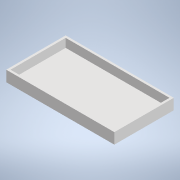
# Autodesk Inventor part: LowerHalf
Saved by Autodesk Inventor 2022 (Build 260153000, 153)
## iProperties
Created: 2023-09-02
Part Number: LowerHalf
Material: Generic
Document SubType Name: Modeling
Designer: Petr Černý
Density: 1 g/cm^3
Appearance: Default
Author: Petr Černý
Autodesk Inventor part; units mm, degrees
ref_plane "YZ Plane" through (0, 0, 0) normal (1, 0, 0) x (0, 1, 0)
ref_plane "XZ Plane" through (0, 0, 0) normal (0, 1, 0) x (-1, 0, 0)
ref_plane "XY Plane" through (0, 0, 0) normal (0, 0, 1) x (1, 0, 0)
sketch "Sketch1" plane through (0, 0, 0) normal (0, 1, 0) x (-1, 0, 0)
  line L0 (-16.8935, 28.2698) -> (97.1065, 28.2698)
  line L1 (97.1065, 28.2698) -> (97.1065, -26.7302)
  line L2 (97.1065, -26.7302) -> (-16.8935, -26.7302)
  line L3 (-16.8935, -26.7302) -> (-16.8935, 28.2698)
  point P0 (0, 0)
  dimension "d0" = 55
  dimension "d1" = 114
  constraints: 8 end point, 2 parallel, 1 horizontal, 1 perpendicular
  measures "d0" distance of L2.end L0.start
  measures "d1" distance of L1.end L2.end
extrude "Extrusion1" add sketch "Sketch1" along normal blind 16
shell "Shell1" thickness 2 removed faces 1 at (-21.1065, 16, 9.9365)
sketch "Sketch2" plane through (-95.1065, 2, -24.7302) normal (0, 1, 0) x (1, 0, 0)
  line L0 (110, 0) -> (110, -51) projected
  line L1 (110, -51) -> (100, -51)
  line L2 (100, -51) -> (100, -41)
  line L3 (100, -41) -> (110, -41)
  line L4 (110, -41) -> (110, -51)
  line L5 (0, 0) -> (110, 0) projected
  line L6 (110, 0) -> (100, 0)
  line L7 (100, 0) -> (100, -10)
  line L8 (100, -10) -> (110, -10)
  line L9 (110, -10) -> (110, 0)
  line L10 (110, -51) -> (0, -51) projected
  line L11 (70, -51) -> (60, -51)
  line L12 (60, -51) -> (60, -41)
  line L13 (60, -41) -> (70, -41)
  line L14 (70, -41) -> (70, -51)
  line L15 (70, 0) -> (60, 0)
  line L16 (60, 0) -> (60, -10)
  line L17 (60, -10) -> (70, -10)
  line L18 (70, -10) -> (70, 0)
  point P0 (95.1065, -24.7302)
  point P1 (65, -46.55)
  point P2 (65, -4.45)
  point P3 (105, -4.4)
  point P4 (105, -46.5)
  point P5 (110, -41)
  point P6 (100, 0)
  point P7 (70, 0)
  point P8 (60, 0)
  point P9 (60, -51)
  dimension "d5" = 10
  dimension "d6" = 10
  dimension "d7" = 10
  dimension "d8" = 10
  dimension "d9" = 10
  dimension "d10" = 10
  dimension "d11" = 10
  dimension "d12" = 10
  dimension "d13" = 30
  dimension "d14" = 30
  dimension "d15" = 4.45
  dimension "d16" = 42.1
  dimension "d17" = 40
  dimension "d18" = 5
  dimension "d19" = 42.1
  dimension "d32" = 4.5
  constraints: 32 end point, 8 parallel, 4 horizontal, 4 perpendicular, 2 point on line
  measures "d5" distance of L2.end L3.end
  measures "d6" distance of L1.end L2.end
  measures "d7" distance of L8.end L7.end
  measures "d8" distance of L7.end L6.end
  measures "d9" distance of L12.end L13.end
  measures "d10" distance of L11.end L12.end
  measures "d11" distance of L17.end L16.end
  measures "d12" distance of L16.end L15.end
  measures "d13" distance between parallel lines of L14 L2
  measures "d14" distance between parallel lines of L7 L18
  measures "d15" distance from line of L11 point (65, -46.55)
  measures "d16" distance of point (65, -4.45) point (65, -46.55)
  measures "d17" distance of point (105, -46.5) point (65, -46.55)
  measures "d18" distance from line of L0 point (105, -46.5)
  measures "d19" distance of point (105, -4.4) point (105, -46.5)
  measures "d32" distance from line of point (105, -46.5) L10
extrude "Extrusion2" add sketch "Sketch2" along normal blind 2
sketch "Sketch3" plane through (-95.1065, 4, -24.7302) normal (0, 1, 0) x (1, 0, 0)
  line L0 (112, 2) -> (-2, 2) projected
  line L1 (112, -53) -> (112, 2) projected
  line L2 (-2, -53) -> (112, -53) projected
  line L3 (-2, 2) -> (-2, -53) projected
  point P0 (95.1065, -24.7302)
  point P1 (65, -46.55)
  point P2 (65, -4.45)
  point P3 (105, -4.4)
  point P4 (105, -46.5)
  point P5 (65, -46.55)
  point P6 (65, -4.45)
  point P7 (105, -46.5)
  point P8 (105, -4.4)
  dimension "d29" = 42.1
  dimension "d30" = 42.1
  dimension "d31" = 40
  constraints: 4 coincident
  measures "d29" distance of point (65, -4.45) point (65, -46.55)
  measures "d30" distance of point (105, -4.4) point (105, -46.5)
  measures "d31" distance of point (65, -46.55) point (105, -46.5)
hole "Hole1" at (-30.1065, 4, 21.8198) at (-30.1065, 4, -20.2802) at (9.8935, 4, -20.3302) at (9.8935, 4, 21.7698) direction (0, -1, 0) diameter 2.459 depth 8.8 tip angle 118 thread size "M3x0.5" class "6H" standard "ISO Metric profile"
sketch "Sketch4" plane through (-97.1065, 0, 28.2698) normal (0, 0, 1) x (1, 0, 0)
  line L0 (72, 16.1171) -> (72, 6.1171) projected
  circle A0 centre (75.47, 8.6194) radius 2.45 projected
  circle A1 centre (85.27, 8.6194) radius 2.45 projected
  circle A2 centre (75.47, 8.6194) radius 2.45
  circle A3 centre (85.27, 8.6194) radius 2.45
  point P0 (97.1065, 0)
  constraints: 2 centre point, 2 coincident, 2 concentric
hole "Hole2" at (-21.6365, 8.6194, 28.2698) at (-11.8365, 8.6194, 28.2698) direction (0, 0, -1) diameter 4.9 depth 2
sketch "Sketch5" plane through (16.8935, 0, 28.2698) normal (1, 0, 0) x (0, 0, -1)
  line L0 (12.5592, 9.5581) -> (21.5731, 9.5581)
  line L1 (21.5731, 9.5581) -> (21.5731, 5.0512)
  line L2 (21.5731, 5.0512) -> (12.5592, 5.0512)
  line L3 (12.5592, 5.0512) -> (12.5592, 9.5581)
  point P0 (28.2698, 0)
  constraints: 8 end point, 2 parallel, 1 horizontal, 1 perpendicular
extrude "Extrusion3" cut sketch "Sketch5" against normal blind 2
body "Solid1"
